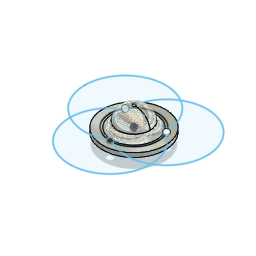
PecaTOF (Autodesk Fusion 360 archive; units mm, degrees)
design "RollerBacl"
Autodesk Fusion 360 part; units mm, degrees
sketch "Sketch1" plane through (0, 0, 0) normal (0, 1, 0) x (1, 0, 0)
  circle A0 centre (0, 0) radius 13
  circle A1 centre (0, 0) radius 21.25
  dimension "d1" = 26
  dimension "d2" = 42.5
  constraint coincident A0.centre A1.centre
  measures "d1" diameter of A0
  measures "d2" diameter of A1
extrude "Extrude1" add sketch "Sketch1" against normal blind 7 contours A0
extrude "Extrude2" add sketch "Sketch1" along normal blind 2.8 contours A0 | A1
sketch "Sketch2" plane through (0, 2.8, 0) normal (0, 1, 0) x (-1, 0, 0)
  circle A0 centre (0, 0) radius 21.25
  circle A1 centre (0, 0) radius 11
  dimension "d7" = 22
  constraint coincident A0.centre A1.centre
  measures "d7" diameter of A1
extrude "Extrude3" add sketch "Sketch2" along normal blind 13 contours A1
fillet "Fillet1" radius 4 1 edges at (10.2556, 2.8, 3.9778)
fillet "Fillet2" radius 10 1 edges at (10.2556, 15.8, -3.9778)
fillet "Fillet3" radius 2 1 edges at (-12.1203, 0, 4.701)
fillet "Fillet4" radius 2 1 edges at (-12.1203, -7, -4.701)
sketch "Sketch3" plane through (0, 2.8, 0) normal (0, 1, 0) x (-1, 0, 0)
  circle A0 centre (0, 0) radius 21.25
  circle A1 centre (0, 0) radius 15
  circle A2 centre (0, 0) radius 16.25
  circle A3 centre (0, 16.25) radius 1.6
  circle A4 centre (-14.0729, -8.125) radius 1.6
  circle A5 centre (14.0729, -8.125) radius 1.6
  circle A6 centre (0, 16.25) radius 27.5
  circle A7 centre (-14.0729, -8.125) radius 27.5
  circle A8 centre (14.0729, -8.125) radius 27.5
  dimension "d18" = 32.5
  dimension "d19" = 3.2
  dimension "d21" = 360
  dimension "d24" = 55
  dimension "d25" = 55
  dimension "d26" = 55
  constraint coincident A0.centre A1.centre
  constraint coincident A2 A3.centre
  constraint concentric A3 A6
  constraint concentric A4 A7
  constraint concentric A5 A8
  measures "d18" diameter of A2
  measures "d19" diameter of A3
  measures "d24" diameter of A6
  measures "d25" diameter of A7
  measures "d26" diameter of A8
extrude "Extrude4" cut sketch "Sketch3" against normal blind 5 contours A2 A3 A7 A8 | A2 A3 A8 | A2 A5 A6 | A2 A5 A6 A7 | A2 A3 A7 | A2 A7 A8 | A1 A2 A3 A7 A8 | A2 A5 A7 | A1 A2 A5 A6 A7 | A2 A6 A7 | A2 A4 A6 A8 | A2 A4 A6 | A1 A2 A3 A7 A8 | A1 A7 A8 | A2 A4 A8 | A1 A2 A5 A6 A7 | A1 A5 A7 | A1 A6 A7 | A1 A2 A4 A6 A8 | A2 A6 A8 | A1 A3 A8 | A1 A3 A7 | A1 A3 A7 A8 | A1 A2 A4 A6 A8 | A1 A5 A6 | A1 A5 A6 A7 | A1 A4 A8 | A1 A6 A8 | A1 A4 A6 | A1 A4 A6 A8
equation "d18 = 42.500 mm - 10 mm"
equation "d24 = 27.5 * 2 mm"
equation "d25 = ( 27.5 * 2 ) * 1 mm"
equation "d26 = ( 27.5 * 2 ) * 1 mm"
